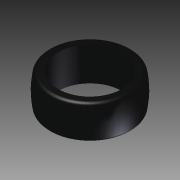
# Autodesk Inventor part: CHAMJ-E50-Rwheel
Saved by Autodesk Inventor 2015 (Build 190159000, 159)
## iProperties
Category: PARTsolutions
Company: MISUMI
Created: 2015-12-24
Part Number: CHAMJ-E50-Rwheel
Catalog Web Link: www.cadenas.de
Description: CHAMJ_E, CHAMK_E, CHAMS_Ewheel-Caster
Vendor: MISUMI
Document SubType Name: Modeling
Designer: psAdmin
Manufacturer: MISUMI
Mass: 15.3195 g
Surface Area: 66.728 cm^2
Volume: 15.3195 cm^3
Density: 1 g/cm^3
Material: 一般
Appearance: PSOLRGB-0-0-0
PSOL_IDENT_0: {$CADENAS_DATA\23d-libs\misumi\metric\42_casters_leveling_pads\chamj_e_wheel.prj},207 {VTYP=3D},{NB=
PSOL_IDENT_1: CHAMJ-E50-Rwheel},{LINA=CHAMJ-E50-Rwheel},{NN=CHAMJ_E, CHAMK_E, CHAMS_Ewheel},{DATE=05.06.2015 05:25
PSOL_IDENT_2: :13},{GEOMDATE=03.09.2009 00:00:00},{VERSION=},{LINEID=30},{LINESUBID=-1},{WBVAR=TSMB,MATW}  {NB=CHA
PSOL_IDENT_3: MJ-E50-Rwheel},{LINA=CHAMJ-E50-Rwheel},{KT=DUMMY},{PN=CHAMJ-E50-R},{TYPE=CHAMJ-E},{TSMB=1},{MATMB=Lo
PSOL_IDENT_4: w Carbon Steel},{STMB=Trivalnt Chromate},{D=50},{MATW=R},{COLORW=Black},{BSP=Available},{BWP=Not Ava
PSOL_IDENT_5: ilable},{H=65},{A=70},{C=42},{F1=56},{F2=28},{DD=6.5},{E=22},{RR=47},{B=20},{TT=2.0},{BR=20},{BU=21}
PSOL_IDENT_6: ,{BN=21},{AL=300},{ALR=300},{ALU=380},{ALN=400},{MASS=180},{COLOR=0.00,0.00,0.00,0.00}
NN: CHAMJ_E, CHAMK_E, CHAMS_Ewheel
NT: Caster
NB: CHAMJ-E50-Rwheel
NBSYN: $PN.wheel
LINA: CHAMJ-E50-Rwheel
TSMB: Swivel
MATMB: Low Carbon Steel
STMB: Trivalnt Chromate
D: 50
MATW: Synthetic Rubber
BSP: Available
BWP: Not Available
H: 65
A: 70
C: 42
F1: 56
F2: 28
DD: 6.5
TT: 2.0
BR: 20
BU: 21
BN: 21
ALR: 300
ALU: 380
ALN: 400
SUPPLIER: MISUMI
ARTICLENO: CHAMJ-E50-Rwheel
BOMINFO: CHAMJ-E50-Rwheel
CREATOR: CADENAS GmbH
Title: CHAMJ-E50-Rwheel
Author: Cadenas PARTsolutions
Comments: Caster
Autodesk Inventor part; units mm, degrees
sketch "Sketch_1" plane through (0, 0, 0) normal (1, 0, 0) x (0, 1, 0)
  line L0 (0, -10) -> (0, 10)
  line L1 (22.2832, 10) -> (19, 10)
  line L2 (19, 10) -> (19, -10)
  line L3 (19, -10) -> (22.2832, -10)
  arc A0 (22.2832, -10) -> (24.2513, -8.3556) centre (22.2832, -8) ccw
  arc A1 (24.2513, -8.3556) -> (24.2513, 8.3556) centre (-22, 0) ccw
  arc A2 (24.2513, 8.3556) -> (22.2832, 10) centre (22.2832, 8) ccw
  constraints: 8 end point, 6 point on circle, 3 centre point
revolve "Revolution1" add sketch "Sketch_1" angle 360 about axis through (0, 0, -10) along (0, 0, -1)
ref_plane "to_bearing_XY" through (0, 0, 0) normal (0, 0, 1) x (1, 0, 0)
ref_plane "to_bearing_YZ" through (0, 0, 0) normal (1, 0, 0) x (0, 1, 0)
ref_plane "to_bearing_ZX" through (0, 0, 0) normal (0, 1, 0) x (0, 0, 1)
body "Solid1"
